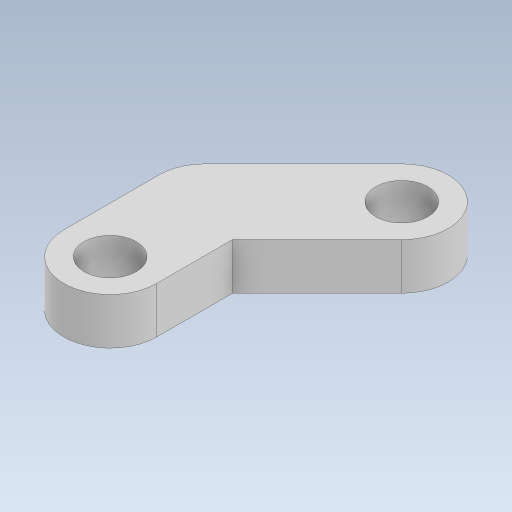
# Autodesk Inventor part: Tensioner
Saved by Autodesk Inventor 2023 (Build 270158000, 158)
## iProperties
Created: 2022-09-14
Part Number: Tensioner
Material: Generic
Document SubType Name: Modeling
Designer: Dave
Density: 1 g/cm^3
Appearance: Default
Author: Dave
Autodesk Inventor part; units mm, degrees
ref_plane "YZ Plane" through (0, 0, 0) normal (1, 0, 0) x (0, 1, 0)
ref_plane "XZ Plane" through (0, 0, 0) normal (0, 1, 0) x (-1, 0, 0)
ref_plane "XY Plane" through (0, 0, 0) normal (0, 0, 1) x (1, 0, 0)
sketch "Sketch1" plane through (0, 0, 0) normal (0, 1, 0) x (-1, 0, 0)
  arc A0 (6, 0) -> (-6, 0) centre (0, 0) ccw
  line L0 (6, 0) -> (6, -12.3)
  line L1 (4.2426, -16.5426) -> (-8.4574, -29.2426)
  line L2 (-16.9426, -20.7574) -> (-6, -9.8147)
  line L3 (-6, -9.8147) -> (-6, 0)
  arc A1 (-16.9426, -20.7574) -> (-8.4574, -29.2426) centre (-12.7, -25) ccw
  arc A2 (4.2426, -16.5426) -> (6, -12.3) centre (0, -12.3) ccw
  point P0 (6, -14.7853)
  dimension "d0" = 12
  dimension "d1" = 12.7
  dimension "d2" = 25
  dimension "d3" = 135
  dimension "d6" = 6
  constraints: 8 end point, 6 point on circle, 6 tangent, 3 centre point, 2 parallel, 2 point on line, 1 coincident, 1 equal radius, 1 vertical
  measures "d0" diameter of A0
  measures "d1" horizontal distance of point (0, 0) A1.centre
  measures "d2" vertical distance of A1.centre point (0, 0)
  measures "d3" angle of L3 L2
  measures "d6" radius of A2
extrude "Extrusion1" add sketch "Sketch1" along normal blind 6
sketch "Sketch2" plane through (0, 6, 0) normal (0, 1, 0) x (1, 0, 0)
  arc A0 (16.9426, 20.7574) -> (8.4574, 29.2426) centre (12.7, 25) ccw projected
  point P0 (0, 0)
hole "Hole1" at (0, 6, 0) at (12.7, 6, -25) direction (0, -1, 0) diameter 6.7564 depth 12.7 tip angle 118 clearance for "Flat Head Machine Screw (82)" size "1/4" standard "Ansi Unified Screw Threads"
body "Solid1"
